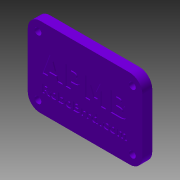
# Autodesk Inventor part: apmb_v1
Saved by Autodesk Inventor 2014 SP1 (Build 180222100, 222)
## iProperties
Created: 2014-02-28
Part Number: apmb_v1
Material: Generic
Document SubType Name: Modeling
Designer: Erin
Density: 1 g/cm^3
Appearance: Default
Author: Erin
Autodesk Inventor part; units mm, degrees
(part 1 of 13)
ref_plane "YZ Plane" through (0, 0, 0) normal (1, 0, 0) x (0, 1, 0)
ref_plane "XY Plane" through (0, 0, 0) normal (0, 0, 1) x (1, 0, 0)
sketch "Sketch1" plane through (0, 0, 0) normal (0, 1, 0) x (-1, 0, 0)
  line L0 (33.3312, 2.2987) -> (35.2468, 0.3832)
  line L1 (20.6882, 2.2987) -> (33.3312, 2.2987)
  line L2 (35.2468, 0.3832) -> (37.29, 0.3832)
  line L3 (22.987, 7.6623) -> (20.0497, 10.5996)
  line L4 (22.987, 2.2987) -> (22.987, 7.6623)
  line L5 (18.7727, 0.3832) -> (20.6882, 2.2987)
  line L6 (16.8571, 0.3832) -> (18.7727, 0.3832)
  line L7 (33.3312, 10.5996) -> (34.7358, 10.5996)
  line L8 (31.1601, 12.7705) -> (33.3312, 10.5996)
  spline S0 degree 3 poles (10.1653, 33.5866) (10.1653, 34.1226) (9.7308, 34.5571) (9.1948, 34.5571) knots 0 0 0 0 1 1 1 1
  line L9 (10.1653, 33.5866) -> (10.1653, 34.1226) construction
  line L10 (10.1653, 34.1226) -> (9.7308, 34.5571) construction
  line L11 (9.7308, 34.5571) -> (9.1948, 34.5571) construction
  spline S1 degree 3 poles (9.1948, 34.5571) (8.6588, 34.5571) (8.2242, 34.1226) (8.2242, 33.5866) knots 0 0 0 0 1 1 1 1
  line L12 (9.1948, 34.5571) -> (8.6588, 34.5571) construction
  line L13 (8.6588, 34.5571) -> (8.2242, 34.1226) construction
  line L14 (8.2242, 34.1226) -> (8.2242, 33.5866) construction
  spline S2 degree 3 poles (8.2242, 33.5866) (8.2242, 33.0506) (8.6588, 32.616) (9.1948, 32.616) knots 0 0 0 0 1 1 1 1
  line L15 (8.2242, 33.5866) -> (8.2242, 33.0506) construction
  line L16 (8.2242, 33.0506) -> (8.6588, 32.616) construction
  line L17 (8.6588, 32.616) -> (9.1948, 32.616) construction
  spline S3 degree 3 poles (9.1948, 32.616) (9.7308, 32.616) (10.1653, 33.0506) (10.1653, 33.5866) knots 0 0 0 0 1 1 1 1
  line L18 (9.1948, 32.616) -> (9.7308, 32.616) construction
  line L19 (9.7308, 32.616) -> (10.1653, 33.0506) construction
  line L20 (10.1653, 33.0506) -> (10.1653, 33.5866) construction
  spline S4 degree 3 poles (12.7194, 33.5866) (12.7194, 34.1226) (12.2849, 34.5571) (11.7489, 34.5571) knots 0 0 0 0 1 1 1 1
  line L21 (12.7194, 33.5866) -> (12.7194, 34.1226) construction
  line L22 (12.7194, 34.1226) -> (12.2849, 34.5571) construction
  line L23 (12.2849, 34.5571) -> (11.7489, 34.5571) construction
  spline S5 degree 3 poles (11.7489, 34.5571) (11.2129, 34.5571) (10.7783, 34.1226) (10.7783, 33.5866) knots 0 0 0 0 1 1 1 1
  line L24 (11.7489, 34.5571) -> (11.2129, 34.5571) construction
  line L25 (11.2129, 34.5571) -> (10.7783, 34.1226) construction
  line L26 (10.7783, 34.1226) -> (10.7783, 33.5866) construction
  spline S6 degree 3 poles (10.7783, 33.5866) (10.7783, 33.0506) (11.2129, 32.616) (11.7489, 32.616) knots 0 0 0 0 1 1 1 1
  line L27 (10.7783, 33.5866) -> (10.7783, 33.0506) construction
  line L28 (10.7783, 33.0506) -> (11.2129, 32.616) construction
  line L29 (11.2129, 32.616) -> (11.7489, 32.616) construction
  spline S7 degree 3 poles (11.7489, 32.616) (12.2849, 32.616) (12.7194, 33.0506) (12.7194, 33.5866) knots 0 0 0 0 1 1 1 1
  line L30 (11.7489, 32.616) -> (12.2849, 32.616) construction
  line L31 (12.2849, 32.616) -> (12.7194, 33.0506) construction
  line L32 (12.7194, 33.0506) -> (12.7194, 33.5866) construction
  spline S8 degree 3 poles (15.2735, 33.5866) (15.2735, 34.1226) (14.839, 34.5571) (14.303, 34.5571) knots 0 0 0 0 1 1 1 1
  line L33 (15.2735, 33.5866) -> (15.2735, 34.1226) construction
  line L34 (15.2735, 34.1226) -> (14.839, 34.5571) construction
  line L35 (14.839, 34.5571) -> (14.303, 34.5571) construction
  spline S9 degree 3 poles (14.303, 34.5571) (13.767, 34.5571) (13.3324, 34.1226) (13.3324, 33.5866) knots 0 0 0 0 1 1 1 1
  line L36 (14.303, 34.5571) -> (13.767, 34.5571) construction
  line L37 (13.767, 34.5571) -> (13.3324, 34.1226) construction
  line L38 (13.3324, 34.1226) -> (13.3324, 33.5866) construction
  spline S10 degree 3 poles (13.3324, 33.5866) (13.3324, 33.0506) (13.767, 32.616) (14.303, 32.616) knots 0 0 0 0 1 1 1 1
  line L39 (13.3324, 33.5866) -> (13.3324, 33.0506) construction
  line L40 (13.3324, 33.0506) -> (13.767, 32.616) construction
  line L41 (13.767, 32.616) -> (14.303, 32.616) construction
  spline S11 degree 3 poles (14.303, 32.616) (14.839, 32.616) (15.2735, 33.0506) (15.2735, 33.5866) knots 0 0 0 0 1 1 1 1
  line L42 (14.303, 32.616) -> (14.839, 32.616) construction
  line L43 (14.839, 32.616) -> (15.2735, 33.0506) construction
  line L44 (15.2735, 33.0506) -> (15.2735, 33.5866) construction
  spline S12 degree 3 poles (17.8276, 23.3701) (17.8276, 23.9061) (17.3931, 24.3407) (16.8571, 24.3407) knots 0 0 0 0 1 1 1 1
  line L45 (17.8276, 23.3701) -> (17.8276, 23.9061) construction
  line L46 (17.8276, 23.9061) -> (17.3931, 24.3407) construction
  line L47 (17.3931, 24.3407) -> (16.8571, 24.3407) construction
  spline S13 degree 3 poles (16.8571, 24.3407) (16.3211, 24.3407) (15.8866, 23.9061) (15.8866, 23.3701) knots 0 0 0 0 1 1 1 1
  line L48 (16.8571, 24.3407) -> (16.3211, 24.3407) construction
  line L49 (16.3211, 24.3407) -> (15.8866, 23.9061) construction
  line L50 (15.8866, 23.9061) -> (15.8866, 23.3701) construction
  spline S14 degree 3 poles (15.8866, 23.3701) (15.8866, 22.8341) (16.3211, 22.3996) (16.8571, 22.3996) knots 0 0 0 0 1 1 1 1
  line L51 (15.8866, 23.3701) -> (15.8866, 22.8341) construction
  line L52 (15.8866, 22.8341) -> (16.3211, 22.3996) construction
  line L53 (16.3211, 22.3996) -> (16.8571, 22.3996) construction
  spline S15 degree 3 poles (16.8571, 22.3996) (17.3931, 22.3996) (17.8276, 22.8341) (17.8276, 23.3701) knots 0 0 0 0 1 1 1 1
  line L54 (16.8571, 22.3996) -> (17.3931, 22.3996) construction
  line L55 (17.3931, 22.3996) -> (17.8276, 22.8341) construction
  line L56 (17.8276, 22.8341) -> (17.8276, 23.3701) construction
  spline S16 degree 3 poles (23.319, 22.2718) (23.319, 22.8078) (22.8844, 23.2424) (22.3485, 23.2424) knots 0 0 0 0 1 1 1 1
  line L57 (23.319, 22.2718) -> (23.319, 22.8078) construction
  line L58 (23.319, 22.8078) -> (22.8844, 23.2424) construction
  line L59 (22.8844, 23.2424) -> (22.3485, 23.2424) construction
  spline S17 degree 3 poles (22.3485, 23.2424) (21.8125, 23.2424) (21.3779, 22.8078) (21.3779, 22.2718) knots 0 0 0 0 1 1 1 1
  line L60 (22.3485, 23.2424) -> (21.8125, 23.2424) construction
  line L61 (21.8125, 23.2424) -> (21.3779, 22.8078) construction
  line L62 (21.3779, 22.8078) -> (21.3779, 22.2718) construction
  spline S18 degree 3 poles (21.3779, 22.2718) (21.3779, 21.7358) (21.8125, 21.3013) (22.3485, 21.3013) knots 0 0 0 0 1 1 1 1
  line L63 (21.3779, 22.2718) -> (21.3779, 21.7358) construction
  line L64 (21.3779, 21.7358) -> (21.8125, 21.3013) construction
  line L65 (21.8125, 21.3013) -> (22.3485, 21.3013) construction
  spline S19 degree 3 poles (22.3485, 21.3013) (22.8844, 21.3013) (23.319, 21.7358) (23.319, 22.2718) knots 0 0 0 0 1 1 1 1
  line L66 (22.3485, 21.3013) -> (22.8844, 21.3013) construction
  line L67 (22.8844, 21.3013) -> (23.319, 21.7358) construction
  line L68 (23.319, 21.7358) -> (23.319, 22.2718) construction
  spline S20 degree 3 poles (25.8731, 22.2718) (25.8731, 22.8078) (25.4385, 23.2424) (24.9026, 23.2424) knots 0 0 0 0 1 1 1 1
  line L69 (25.8731, 22.2718) -> (25.8731, 22.8078) construction
  line L70 (25.8731, 22.8078) -> (25.4385, 23.2424) construction
  line L71 (25.4385, 23.2424) -> (24.9026, 23.2424) construction
  spline S21 degree 3 poles (24.9026, 23.2424) (24.3666, 23.2424) (23.932, 22.8078) (23.932, 22.2718) knots 0 0 0 0 1 1 1 1
  line L72 (24.9026, 23.2424) -> (24.3666, 23.2424) construction
  line L73 (24.3666, 23.2424) -> (23.932, 22.8078) construction
  line L74 (23.932, 22.8078) -> (23.932, 22.2718) construction
  spline S22 degree 3 poles (23.932, 22.2718) (23.932, 21.7358) (24.3666, 21.3013) (24.9026, 21.3013) knots 0 0 0 0 1 1 1 1
  line L75 (23.932, 22.2718) -> (23.932, 21.7358) construction
  line L76 (23.932, 21.7358) -> (24.3666, 21.3013) construction
  line L77 (24.3666, 21.3013) -> (24.9026, 21.3013) construction
  spline S23 degree 3 poles (24.9026, 21.3013) (25.4385, 21.3013) (25.8731, 21.7358) (25.8731, 22.2718) knots 0 0 0 0 1 1 1 1
  line L78 (24.9026, 21.3013) -> (25.4385, 21.3013) construction
  line L79 (25.4385, 21.3013) -> (25.8731, 21.7358) construction
  line L80 (25.8731, 21.7358) -> (25.8731, 22.2718) construction
  spline S24 degree 3 poles (23.319, 24.8259) (23.319, 25.3619) (22.8844, 25.7965) (22.3485, 25.7965) knots 0 0 0 0 1 1 1 1
  line L81 (23.319, 24.8259) -> (23.319, 25.3619) construction
  line L82 (23.319, 25.3619) -> (22.8844, 25.7965) construction
  line L83 (22.8844, 25.7965) -> (22.3485, 25.7965) construction
  spline S25 degree 3 poles (22.3485, 25.7965) (21.8125, 25.7965) (21.3779, 25.3619) (21.3779, 24.8259) knots 0 0 0 0 1 1 1 1
  line L84 (22.3485, 25.7965) -> (21.8125, 25.7965) construction
  line L85 (21.8125, 25.7965) -> (21.3779, 25.3619) construction
  line L86 (21.3779, 25.3619) -> (21.3779, 24.8259) construction
  spline S26 degree 3 poles (21.3779, 24.8259) (21.3779, 24.2899) (21.8125, 23.8554) (22.3485, 23.8554) knots 0 0 0 0 1 1 1 1
  line L87 (21.3779, 24.8259) -> (21.3779, 24.2899) construction
  line L88 (21.3779, 24.2899) -> (21.8125, 23.8554) construction
  line L89 (21.8125, 23.8554) -> (22.3485, 23.8554) construction
  spline S27 degree 3 poles (22.3485, 23.8554) (22.8844, 23.8554) (23.319, 24.2899) (23.319, 24.8259) knots 0 0 0 0 1 1 1 1
  line L90 (22.3485, 23.8554) -> (22.8844, 23.8554) construction
  line L91 (22.8844, 23.8554) -> (23.319, 24.2899) construction
  line L92 (23.319, 24.2899) -> (23.319, 24.8259) construction
  spline S28 degree 3 poles (25.8731, 24.8259) (25.8731, 25.3619) (25.4385, 25.7965) (24.9026, 25.7965) knots 0 0 0 0 1 1 1 1
  line L93 (25.8731, 24.8259) -> (25.8731, 25.3619) construction
  line L94 (25.8731, 25.3619) -> (25.4385, 25.7965) construction
  line L95 (25.4385, 25.7965) -> (24.9026, 25.7965) construction
  spline S29 degree 3 poles (24.9026, 25.7965) (24.3666, 25.7965) (23.932, 25.3619) (23.932, 24.8259) knots 0 0 0 0 1 1 1 1
  line L96 (24.9026, 25.7965) -> (24.3666, 25.7965) construction
  line L97 (24.3666, 25.7965) -> (23.932, 25.3619) construction
  line L98 (23.932, 25.3619) -> (23.932, 24.8259) construction
  spline S30 degree 3 poles (23.932, 24.8259) (23.932, 24.2899) (24.3666, 23.8554) (24.9026, 23.8554) knots 0 0 0 0 1 1 1 1
  line L99 (23.932, 24.8259) -> (23.932, 24.2899) construction
  line L100 (23.932, 24.2899) -> (24.3666, 23.8554) construction
  line L101 (24.3666, 23.8554) -> (24.9026, 23.8554) construction
  spline S31 degree 3 poles (24.9026, 23.8554) (25.4385, 23.8554) (25.8731, 24.2899) (25.8731, 24.8259) knots 0 0 0 0 1 1 1 1
  line L102 (24.9026, 23.8554) -> (25.4385, 23.8554) construction
  line L103 (25.4385, 23.8554) -> (25.8731, 24.2899) construction
  line L104 (25.8731, 24.2899) -> (25.8731, 24.8259) construction
  spline S32 degree 3 poles (20.3818, 23.3701) (20.3818, 23.9061) (19.9472, 24.3407) (19.4112, 24.3407) knots 0 0 0 0 1 1 1 1
  line L105 (20.3818, 23.3701) -> (20.3818, 23.9061) construction
  line L106 (20.3818, 23.9061) -> (19.9472, 24.3407) construction
  line L107 (19.9472, 24.3407) -> (19.4112, 24.3407) construction
  spline S33 degree 3 poles (19.4112, 24.3407) (18.8752, 24.3407) (18.4407, 23.9061) (18.4407, 23.3701) knots 0 0 0 0 1 1 1 1
  line L108 (19.4112, 24.3407) -> (18.8752, 24.3407) construction
  line L109 (18.8752, 24.3407) -> (18.4407, 23.9061) construction
  line L110 (18.4407, 23.9061) -> (18.4407, 23.3701) construction
  spline S34 degree 3 poles (18.4407, 23.3701) (18.4407, 22.8341) (18.8752, 22.3996) (19.4112, 22.3996) knots 0 0 0 0 1 1 1 1
  line L111 (18.4407, 23.3701) -> (18.4407, 22.8341) construction
  line L112 (18.4407, 22.8341) -> (18.8752, 22.3996) construction
  line L113 (18.8752, 22.3996) -> (19.4112, 22.3996) construction
  spline S35 degree 3 poles (19.4112, 22.3996) (19.9472, 22.3996) (20.3818, 22.8341) (20.3818, 23.3701) knots 0 0 0 0 1 1 1 1
  line L114 (19.4112, 22.3996) -> (19.9472, 22.3996) construction
  line L115 (19.9472, 22.3996) -> (20.3818, 22.8341) construction
  line L116 (20.3818, 22.8341) -> (20.3818, 23.3701) construction
  spline S36 degree 3 poles (20.3818, 25.9242) (20.3818, 26.4602) (19.9472, 26.8948) (19.4112, 26.8948) knots 0 0 0 0 1 1 1 1
  line L117 (20.3818, 25.9242) -> (20.3818, 26.4602) construction
  line L118 (20.3818, 26.4602) -> (19.9472, 26.8948) construction
  line L119 (19.9472, 26.8948) -> (19.4112, 26.8948) construction
  spline S37 degree 3 poles (19.4112, 26.8948) (18.8752, 26.8948) (18.4407, 26.4602) (18.4407, 25.9242) knots 0 0 0 0 1 1 1 1
  line L120 (19.4112, 26.8948) -> (18.8752, 26.8948) construction
  line L121 (18.8752, 26.8948) -> (18.4407, 26.4602) construction
  line L122 (18.4407, 26.4602) -> (18.4407, 25.9242) construction
  spline S38 degree 3 poles (18.4407, 25.9242) (18.4407, 25.3882) (18.8752, 24.9537) (19.4112, 24.9537) knots 0 0 0 0 1 1 1 1
  line L123 (18.4407, 25.9242) -> (18.4407, 25.3882) construction
  line L124 (18.4407, 25.3882) -> (18.8752, 24.9537) construction
  line L125 (18.8752, 24.9537) -> (19.4112, 24.9537) construction
  spline S39 degree 3 poles (19.4112, 24.9537) (19.9472, 24.9537) (20.3818, 25.3882) (20.3818, 25.9242) knots 0 0 0 0 1 1 1 1
  line L126 (19.4112, 24.9537) -> (19.9472, 24.9537) construction
  line L127 (19.9472, 24.9537) -> (20.3818, 25.3882) construction
  line L128 (20.3818, 25.3882) -> (20.3818, 25.9242) construction
  spline S40 degree 3 poles (20.3818, 28.4784) (20.3818, 29.0143) (19.9472, 29.4489) (19.4112, 29.4489) knots 0 0 0 0 1 1 1 1
  line L129 (20.3818, 28.4784) -> (20.3818, 29.0143) construction
  line L130 (20.3818, 29.0143) -> (19.9472, 29.4489) construction
  line L131 (19.9472, 29.4489) -> (19.4112, 29.4489) construction
  spline S41 degree 3 poles (19.4112, 29.4489) (18.8752, 29.4489) (18.4407, 29.0143) (18.4407, 28.4784) knots 0 0 0 0 1 1 1 1
  line L132 (19.4112, 29.4489) -> (18.8752, 29.4489) construction
  line L133 (18.8752, 29.4489) -> (18.4407, 29.0143) construction
  line L134 (18.4407, 29.0143) -> (18.4407, 28.4784) construction
  spline S42 degree 3 poles (18.4407, 28.4784) (18.4407, 27.9423) (18.8752, 27.5078) (19.4112, 27.5078) knots 0 0 0 0 1 1 1 1
  line L135 (18.4407, 28.4784) -> (18.4407, 27.9423) construction
  line L136 (18.4407, 27.9423) -> (18.8752, 27.5078) construction
  line L137 (18.8752, 27.5078) -> (19.4112, 27.5078) construction
  spline S43 degree 3 poles (19.4112, 27.5078) (19.9472, 27.5078) (20.3818, 27.9423) (20.3818, 28.4784) knots 0 0 0 0 1 1 1 1
  line L138 (19.4112, 27.5078) -> (19.9472, 27.5078) construction
  line L139 (19.9472, 27.5078) -> (20.3818, 27.9423) construction
  line L140 (20.3818, 27.9423) -> (20.3818, 28.4784) construction
  spline S44 degree 3 poles (20.3818, 31.0325) (20.3818, 31.5684) (19.9472, 32.003) (19.4112, 32.003) knots 0 0 0 0 1 1 1 1
  line L141 (20.3818, 31.0325) -> (20.3818, 31.5684) construction
  line L142 (20.3818, 31.5684) -> (19.9472, 32.003) construction
  line L143 (19.9472, 32.003) -> (19.4112, 32.003) construction
  spline S45 degree 3 poles (19.4112, 32.003) (18.8752, 32.003) (18.4407, 31.5684) (18.4407, 31.0325) knots 0 0 0 0 1 1 1 1
  line L144 (19.4112, 32.003) -> (18.8752, 32.003) construction
  line L145 (18.8752, 32.003) -> (18.4407, 31.5684) construction
  line L146 (18.4407, 31.5684) -> (18.4407, 31.0325) construction
  spline S46 degree 3 poles (18.4407, 31.0325) (18.4407, 30.4965) (18.8752, 30.0619) (19.4112, 30.0619) knots 0 0 0 0 1 1 1 1
  line L147 (18.4407, 31.0325) -> (18.4407, 30.4965) construction
  line L148 (18.4407, 30.4965) -> (18.8752, 30.0619) construction
  line L149 (18.8752, 30.0619) -> (19.4112, 30.0619) construction
  spline S47 degree 3 poles (19.4112, 30.0619) (19.9472, 30.0619) (20.3818, 30.4965) (20.3818, 31.0325) knots 0 0 0 0 1 1 1 1
  line L150 (19.4112, 30.0619) -> (19.9472, 30.0619) construction
  line L151 (19.9472, 30.0619) -> (20.3818, 30.4965) construction
  line L152 (20.3818, 30.4965) -> (20.3818, 31.0325) construction
  spline S48 degree 3 poles (17.8276, 25.9242) (17.8276, 26.4602) (17.3931, 26.8948) (16.8571, 26.8948) knots 0 0 0 0 1 1 1 1
  line L153 (17.8276, 25.9242) -> (17.8276, 26.4602) construction
  line L154 (17.8276, 26.4602) -> (17.3931, 26.8948) construction
  line L155 (17.3931, 26.8948) -> (16.8571, 26.8948) construction
  spline S49 degree 3 poles (16.8571, 26.8948) (16.3211, 26.8948) (15.8866, 26.4602) (15.8866, 25.9242) knots 0 0 0 0 1 1 1 1
  line L156 (16.8571, 26.8948) -> (16.3211, 26.8948) construction
  line L157 (16.3211, 26.8948) -> (15.8866, 26.4602) construction
  line L158 (15.8866, 26.4602) -> (15.8866, 25.9242) construction
  spline S50 degree 3 poles (15.8866, 25.9242) (15.8866, 25.3882) (16.3211, 24.9537) (16.8571, 24.9537) knots 0 0 0 0 1 1 1 1
  line L159 (15.8866, 25.9242) -> (15.8866, 25.3882) construction
  line L160 (15.8866, 25.3882) -> (16.3211, 24.9537) construction
  line L161 (16.3211, 24.9537) -> (16.8571, 24.9537) construction
  spline S51 degree 3 poles (16.8571, 24.9537) (17.3931, 24.9537) (17.8276, 25.3882) (17.8276, 25.9242) knots 0 0 0 0 1 1 1 1
  line L162 (16.8571, 24.9537) -> (17.3931, 24.9537) construction
  line L163 (17.3931, 24.9537) -> (17.8276, 25.3882) construction
  line L164 (17.8276, 25.3882) -> (17.8276, 25.9242) construction
  spline S52 degree 3 poles (17.8276, 28.4784) (17.8276, 29.0143) (17.3931, 29.4489) (16.8571, 29.4489) knots 0 0 0 0 1 1 1 1
  line L165 (17.8276, 28.4784) -> (17.8276, 29.0143) construction
  line L166 (17.8276, 29.0143) -> (17.3931, 29.4489) construction
  line L167 (17.3931, 29.4489) -> (16.8571, 29.4489) construction
  spline S53 degree 3 poles (16.8571, 29.4489) (16.3211, 29.4489) (15.8866, 29.0143) (15.8866, 28.4784) knots 0 0 0 0 1 1 1 1
  line L168 (16.8571, 29.4489) -> (16.3211, 29.4489) construction
  line L169 (16.3211, 29.4489) -> (15.8866, 29.0143) construction
  line L170 (15.8866, 29.0143) -> (15.8866, 28.4784) construction
  spline S54 degree 3 poles (15.8866, 28.4784) (15.8866, 27.9423) (16.3211, 27.5078) (16.8571, 27.5078) knots 0 0 0 0 1 1 1 1
  line L171 (15.8866, 28.4784) -> (15.8866, 27.9423) construction
  line L172 (15.8866, 27.9423) -> (16.3211, 27.5078) construction
  line L173 (16.3211, 27.5078) -> (16.8571, 27.5078) construction
  spline S55 degree 3 poles (16.8571, 27.5078) (17.3931, 27.5078) (17.8276, 27.9423) (17.8276, 28.4784) knots 0 0 0 0 1 1 1 1
  line L174 (16.8571, 27.5078) -> (17.3931, 27.5078) construction
  line L175 (17.3931, 27.5078) -> (17.8276, 27.9423) construction
  line L176 (17.8276, 27.9423) -> (17.8276, 28.4784) construction
  spline S56 degree 3 poles (17.8276, 31.0325) (17.8276, 31.5684) (17.3931, 32.003) (16.8571, 32.003) knots 0 0 0 0 1 1 1 1
  line L177 (17.8276, 31.0325) -> (17.8276, 31.5684) construction
  line L178 (17.8276, 31.5684) -> (17.3931, 32.003) construction
  line L179 (17.3931, 32.003) -> (16.8571, 32.003) construction
  spline S57 degree 3 poles (16.8571, 32.003) (16.3211, 32.003) (15.8866, 31.5684) (15.8866, 31.0325) knots 0 0 0 0 1 1 1 1
  line L180 (16.8571, 32.003) -> (16.3211, 32.003) construction
  line L181 (16.3211, 32.003) -> (15.8866, 31.5684) construction
  line L182 (15.8866, 31.5684) -> (15.8866, 31.0325) construction
  spline S58 degree 3 poles (15.8866, 31.0325) (15.8866, 30.4965) (16.3211, 30.0619) (16.8571, 30.0619) knots 0 0 0 0 1 1 1 1
  line L183 (15.8866, 31.0325) -> (15.8866, 30.4965) construction
  line L184 (15.8866, 30.4965) -> (16.3211, 30.0619) construction
  line L185 (16.3211, 30.0619) -> (16.8571, 30.0619) construction
  spline S59 degree 3 poles (16.8571, 30.0619) (17.3931, 30.0619) (17.8276, 30.4965) (17.8276, 31.0325) knots 0 0 0 0 1 1 1 1
  line L186 (16.8571, 30.0619) -> (17.3931, 30.0619) construction
  line L187 (17.3931, 30.0619) -> (17.8276, 30.4965) construction
  line L188 (17.8276, 30.4965) -> (17.8276, 31.0325) construction
  spline S60 degree 3 poles (38.2606, 33.5866) (38.2606, 34.1226) (37.826, 34.5571) (37.29, 34.5571) knots 0 0 0 0 1 1 1 1
  line L189 (38.2606, 33.5866) -> (38.2606, 34.1226) construction
  line L190 (38.2606, 34.1226) -> (37.826, 34.5571) construction
  line L191 (37.826, 34.5571) -> (37.29, 34.5571) construction
  spline S61 degree 3 poles (37.29, 34.5571) (36.754, 34.5571) (36.3194, 34.1226) (36.3194, 33.5866) knots 0 0 0 0 1 1 1 1
  line L192 (37.29, 34.5571) -> (36.754, 34.5571) construction
  line L193 (36.754, 34.5571) -> (36.3194, 34.1226) construction
  line L194 (36.3194, 34.1226) -> (36.3194, 33.5866) construction
  spline S62 degree 3 poles (36.3194, 33.5866) (36.3194, 33.0506) (36.754, 32.616) (37.29, 32.616) knots 0 0 0 0 1 1 1 1
  line L195 (36.3194, 33.5866) -> (36.3194, 33.0506) construction
  line L196 (36.3194, 33.0506) -> (36.754, 32.616) construction
  line L197 (36.754, 32.616) -> (37.29, 32.616) construction
  spline S63 degree 3 poles (37.29, 32.616) (37.826, 32.616) (38.2606, 33.0506) (38.2606, 33.5866) knots 0 0 0 0 1 1 1 1
  line L198 (37.29, 32.616) -> (37.826, 32.616) construction
  line L199 (37.826, 32.616) -> (38.2606, 33.0506) construction
  line L200 (38.2606, 33.0506) -> (38.2606, 33.5866) construction
  spline S64 degree 3 poles (40.8147, 33.5866) (40.8147, 34.1226) (40.3801, 34.5571) (39.8441, 34.5571) knots 0 0 0 0 1 1 1 1
  line L201 (40.8147, 33.5866) -> (40.8147, 34.1226) construction
  line L202 (40.8147, 34.1226) -> (40.3801, 34.5571) construction
  line L203 (40.3801, 34.5571) -> (39.8441, 34.5571) construction
  spline S65 degree 3 poles (39.8441, 34.5571) (39.3081, 34.5571) (38.8735, 34.1226) (38.8735, 33.5866) knots 0 0 0 0 1 1 1 1
  line L204 (39.8441, 34.5571) -> (39.3081, 34.5571) construction
  line L205 (39.3081, 34.5571) -> (38.8735, 34.1226) construction
  line L206 (38.8735, 34.1226) -> (38.8735, 33.5866) construction
  spline S66 degree 3 poles (38.8735, 33.5866) (38.8735, 33.0506) (39.3081, 32.616) (39.8441, 32.616) knots 0 0 0 0 1 1 1 1
  line L207 (38.8735, 33.5866) -> (38.8735, 33.0506) construction
  line L208 (38.8735, 33.0506) -> (39.3081, 32.616) construction
  line L209 (39.3081, 32.616) -> (39.8441, 32.616) construction
  spline S67 degree 3 poles (39.8441, 32.616) (40.3801, 32.616) (40.8147, 33.0506) (40.8147, 33.5866) knots 0 0 0 0 1 1 1 1
  line L210 (39.8441, 32.616) -> (40.3801, 32.616) construction
  line L211 (40.3801, 32.616) -> (40.8147, 33.0506) construction
  line L212 (40.8147, 33.0506) -> (40.8147, 33.5866) construction
  spline S68 degree 3 poles (43.3688, 33.5866) (43.3688, 34.1226) (42.9342, 34.5571) (42.3982, 34.5571) knots 0 0 0 0 1 1 1 1
  line L213 (43.3688, 33.5866) -> (43.3688, 34.1226) construction
  line L214 (43.3688, 34.1226) -> (42.9342, 34.5571) construction
  line L215 (42.9342, 34.5571) -> (42.3982, 34.5571) construction
  spline S69 degree 3 poles (42.3982, 34.5571) (41.8622, 34.5571) (41.4277, 34.1226) (41.4277, 33.5866) knots 0 0 0 0 1 1 1 1
  line L216 (42.3982, 34.5571) -> (41.8622, 34.5571) construction
  line L217 (41.8622, 34.5571) -> (41.4277, 34.1226) construction
  line L218 (41.4277, 34.1226) -> (41.4277, 33.5866) construction
  spline S70 degree 3 poles (41.4277, 33.5866) (41.4277, 33.0506) (41.8622, 32.616) (42.3982, 32.616) knots 0 0 0 0 1 1 1 1
  line L219 (41.4277, 33.5866) -> (41.4277, 33.0506) construction
  line L220 (41.4277, 33.0506) -> (41.8622, 32.616) construction
  line L221 (41.8622, 32.616) -> (42.3982, 32.616) construction
  spline S71 degree 3 poles (42.3982, 32.616) (42.9342, 32.616) (43.3688, 33.0506) (43.3688, 33.5866) knots 0 0 0 0 1 1 1 1
  line L222 (42.3982, 32.616) -> (42.9342, 32.616) construction
  line L223 (42.9342, 32.616) -> (43.3688, 33.0506) construction
  line L224 (43.3688, 33.0506) -> (43.3688, 33.5866) construction
  spline S72 degree 3 poles (45.9229, 33.5866) (45.9229, 34.1226) (45.4883, 34.5571) (44.9523, 34.5571) knots 0 0 0 0 1 1 1 1
  line L225 (45.9229, 33.5866) -> (45.9229, 34.1226) construction
  line L226 (45.9229, 34.1226) -> (45.4883, 34.5571) construction
  line L227 (45.4883, 34.5571) -> (44.9523, 34.5571) construction
  spline S73 degree 3 poles (44.9523, 34.5571) (44.4163, 34.5571) (43.9818, 34.1226) (43.9818, 33.5866) knots 0 0 0 0 1 1 1 1
  line L228 (44.9523, 34.5571) -> (44.4163, 34.5571) construction
  line L229 (44.4163, 34.5571) -> (43.9818, 34.1226) construction
  line L230 (43.9818, 34.1226) -> (43.9818, 33.5866) construction
  spline S74 degree 3 poles (43.9818, 33.5866) (43.9818, 33.0506) (44.4163, 32.616) (44.9523, 32.616) knots 0 0 0 0 1 1 1 1
  line L231 (43.9818, 33.5866) -> (43.9818, 33.0506) construction
  line L232 (43.9818, 33.0506) -> (44.4163, 32.616) construction
  line L233 (44.4163, 32.616) -> (44.9523, 32.616) construction
  spline S75 degree 3 poles (44.9523, 32.616) (45.4883, 32.616) (45.9229, 33.0506) (45.9229, 33.5866) knots 0 0 0 0 1 1 1 1
  line L234 (44.9523, 32.616) -> (45.4883, 32.616) construction
  line L235 (45.4883, 32.616) -> (45.9229, 33.0506) construction
  line L236 (45.9229, 33.0506) -> (45.9229, 33.5866) construction
  spline S76 degree 3 poles (34.4294, 0.3832) (34.4294, 0.9191) (33.9948, 1.3537) (33.4588, 1.3537) knots 0 0 0 0 1 1 1 1
  line L237 (34.4294, 0.3832) -> (34.4294, 0.9191) construction
  line L238 (34.4294, 0.9191) -> (33.9948, 1.3537) construction
  line L239 (33.9948, 1.3537) -> (33.4588, 1.3537) construction
  spline S77 degree 3 poles (33.4588, 1.3537) (32.9228, 1.3537) (32.4883, 0.9191) (32.4883, 0.3832) knots 0 0 0 0 1 1 1 1
  line L240 (33.4588, 1.3537) -> (32.9228, 1.3537) construction
  line L241 (32.9228, 1.3537) -> (32.4883, 0.9191) construction
  line L242 (32.4883, 0.9191) -> (32.4883, 0.3832) construction
  spline S78 degree 3 poles (32.4883, 0.3832) (32.4883, -0.1529) (32.9228, -0.5874) (33.4588, -0.5874) knots 0 0 0 0 1 1 1 1
  line L243 (32.4883, 0.3832) -> (32.4883, -0.1529) construction
  line L244 (32.4883, -0.1529) -> (32.9228, -0.5874) construction
  line L245 (32.9228, -0.5874) -> (33.4588, -0.5874) construction
  spline S79 degree 3 poles (33.4588, -0.5874) (33.9948, -0.5874) (34.4294, -0.1529) (34.4294, 0.3832) knots 0 0 0 0 1 1 1 1
  line L246 (33.4588, -0.5874) -> (33.9948, -0.5874) construction
  line L247 (33.9948, -0.5874) -> (34.4294, -0.1529) construction
  line L248 (34.4294, -0.1529) -> (34.4294, 0.3832) construction
  spline S80 degree 3 poles (31.8752, 0.3832) (31.8752, 0.9191) (31.4407, 1.3537) (30.9047, 1.3537) knots 0 0 0 0 1 1 1 1
  line L249 (31.8752, 0.3832) -> (31.8752, 0.9191) construction
  line L250 (31.8752, 0.9191) -> (31.4407, 1.3537) construction
  line L251 (31.4407, 1.3537) -> (30.9047, 1.3537) construction
  spline S81 degree 3 poles (30.9047, 1.3537) (30.3687, 1.3537) (29.9342, 0.9191) (29.9342, 0.3832) knots 0 0 0 0 1 1 1 1
  line L252 (30.9047, 1.3537) -> (30.3687, 1.3537) construction
  line L253 (30.3687, 1.3537) -> (29.9342, 0.9191) construction
  line L254 (29.9342, 0.9191) -> (29.9342, 0.3832) construction
  spline S82 degree 3 poles (29.9342, 0.3832) (29.9342, -0.1529) (30.3687, -0.5874) (30.9047, -0.5874) knots 0 0 0 0 1 1 1 1
  line L255 (29.9342, 0.3832) -> (29.9342, -0.1529) construction
  line L256 (29.9342, -0.1529) -> (30.3687, -0.5874) construction
  line L257 (30.3687, -0.5874) -> (30.9047, -0.5874) construction
  spline S83 degree 3 poles (30.9047, -0.5874) (31.4407, -0.5874) (31.8752, -0.1529) (31.8752, 0.3832) knots 0 0 0 0 1 1 1 1
  line L258 (30.9047, -0.5874) -> (31.4407, -0.5874) construction
  line L259 (31.4407, -0.5874) -> (31.8752, -0.1529) construction
  line L260 (31.8752, -0.1529) -> (31.8752, 0.3832) construction
  spline S84 degree 3 poles (29.3211, 0.3832) (29.3211, 0.9191) (28.8866, 1.3537) (28.3506, 1.3537) knots 0 0 0 0 1 1 1 1
  line L261 (29.3211, 0.3832) -> (29.3211, 0.9191) construction
  line L262 (29.3211, 0.9191) -> (28.8866, 1.3537) construction
  line L263 (28.8866, 1.3537) -> (28.3506, 1.3537) construction
  spline S85 degree 3 poles (28.3506, 1.3537) (27.8146, 1.3537) (27.3801, 0.9191) (27.3801, 0.3832) knots 0 0 0 0 1 1 1 1
  line L264 (28.3506, 1.3537) -> (27.8146, 1.3537) construction
  line L265 (27.8146, 1.3537) -> (27.3801, 0.9191) construction
  line L266 (27.3801, 0.9191) -> (27.3801, 0.3832) construction
  spline S86 degree 3 poles (27.3801, 0.3832) (27.3801, -0.1529) (27.8146, -0.5874) (28.3506, -0.5874) knots 0 0 0 0 1 1 1 1
  line L267 (27.3801, 0.3832) -> (27.3801, -0.1529) construction
  line L268 (27.3801, -0.1529) -> (27.8146, -0.5874) construction
  line L269 (27.8146, -0.5874) -> (28.3506, -0.5874) construction
  spline S87 degree 3 poles (28.3506, -0.5874) (28.8866, -0.5874) (29.3211, -0.1529) (29.3211, 0.3832) knots 0 0 0 0 1 1 1 1
  line L270 (28.3506, -0.5874) -> (28.8866, -0.5874) construction
  line L271 (28.8866, -0.5874) -> (29.3211, -0.1529) construction
  line L272 (29.3211, -0.1529) -> (29.3211, 0.3832) construction
  spline S88 degree 3 poles (43.3688, 0.3832) (43.3688, 0.9191) (42.9342, 1.3537) (42.3982, 1.3537) knots 0 0 0 0 1 1 1 1
  line L273 (43.3688, 0.3832) -> (43.3688, 0.9191) construction
  line L274 (43.3688, 0.9191) -> (42.9342, 1.3537) construction
  line L275 (42.9342, 1.3537) -> (42.3982, 1.3537) construction
  spline S89 degree 3 poles (42.3982, 1.3537) (41.8622, 1.3537) (41.4277, 0.9191) (41.4277, 0.3832) knots 0 0 0 0 1 1 1 1
  line L276 (42.3982, 1.3537) -> (41.8622, 1.3537) construction
  line L277 (41.8622, 1.3537) -> (41.4277, 0.9191) construction
  line L278 (41.4277, 0.9191) -> (41.4277, 0.3832) construction
  spline S90 degree 3 poles (41.4277, 0.3832) (41.4277, -0.1529) (41.8622, -0.5874) (42.3982, -0.5874) knots 0 0 0 0 1 1 1 1
  line L279 (41.4277, 0.3832) -> (41.4277, -0.1529) construction
  line L280 (41.4277, -0.1529) -> (41.8622, -0.5874) construction
  line L281 (41.8622, -0.5874) -> (42.3982, -0.5874) construction
  spline S91 degree 3 poles (42.3982, -0.5874) (42.9342, -0.5874) (43.3688, -0.1529) (43.3688, 0.3832) knots 0 0 0 0 1 1 1 1
  line L282 (42.3982, -0.5874) -> (42.9342, -0.5874) construction
  line L283 (42.9342, -0.5874) -> (43.3688, -0.1529) construction
  line L284 (43.3688, -0.1529) -> (43.3688, 0.3832) construction
  spline S92 degree 3 poles (35.7064, 2.9373) (35.7064, 3.4732) (35.2719, 3.9078) (34.7358, 3.9078) knots 0 0 0 0 1 1 1 1
  line L285 (35.7064, 2.9373) -> (35.7064, 3.4732) construction
  line L286 (35.7064, 3.4732) -> (35.2719, 3.9078) construction
  line L287 (35.2719, 3.9078) -> (34.7358, 3.9078) construction
  spline S93 degree 3 poles (34.7358, 3.9078) (34.1999, 3.9078) (33.7653, 3.4732) (33.7653, 2.9373) knots 0 0 0 0 1 1 1 1
  line L288 (34.7358, 3.9078) -> (34.1999, 3.9078) construction
  line L289 (34.1999, 3.9078) -> (33.7653, 3.4732) construction
  line L290 (33.7653, 3.4732) -> (33.7653, 2.9373) construction
  spline S94 degree 3 poles (33.7653, 2.9373) (33.7653, 2.4013) (34.1999, 1.9667) (34.7358, 1.9667) knots 0 0 0 0 1 1 1 1
  line L291 (33.7653, 2.9373) -> (33.7653, 2.4013) construction
  line L292 (33.7653, 2.4013) -> (34.1999, 1.9667) construction
  line L293 (34.1999, 1.9667) -> (34.7358, 1.9667) construction
  spline S95 degree 3 poles (34.7358, 1.9667) (35.2719, 1.9667) (35.7064, 2.4013) (35.7064, 2.9373) knots 0 0 0 0 1 1 1 1
  line L294 (34.7358, 1.9667) -> (35.2719, 1.9667) construction
  line L295 (35.2719, 1.9667) -> (35.7064, 2.4013) construction
  line L296 (35.7064, 2.4013) -> (35.7064, 2.9373) construction
  spline S96 degree 3 poles (35.7064, 5.4914) (35.7064, 6.0273) (35.2719, 6.4619) (34.7358, 6.4619) knots 0 0 0 0 1 1 1 1
  line L297 (35.7064, 5.4914) -> (35.7064, 6.0273) construction
  line L298 (35.7064, 6.0273) -> (35.2719, 6.4619) construction
  line L299 (35.2719, 6.4619) -> (34.7358, 6.4619) construction
  spline S97 degree 3 poles (34.7358, 6.4619) (34.1999, 6.4619) (33.7653, 6.0273) (33.7653, 5.4914) knots 0 0 0 0 1 1 1 1
  line L300 (34.7358, 6.4619) -> (34.1999, 6.4619) construction
  line L301 (34.1999, 6.4619) -> (33.7653, 6.0273) construction
  line L302 (33.7653, 6.0273) -> (33.7653, 5.4914) construction
  spline S98 degree 3 poles (33.7653, 5.4914) (33.7653, 4.9554) (34.1999, 4.5208) (34.7358, 4.5208) knots 0 0 0 0 1 1 1 1
  line L303 (33.7653, 5.4914) -> (33.7653, 4.9554) construction
  line L304 (33.7653, 4.9554) -> (34.1999, 4.5208) construction
  line L305 (34.1999, 4.5208) -> (34.7358, 4.5208) construction
  spline S99 degree 3 poles (34.7358, 4.5208) (35.2719, 4.5208) (35.7064, 4.9554) (35.7064, 5.4914) knots 0 0 0 0 1 1 1 1
  line L306 (34.7358, 4.5208) -> (35.2719, 4.5208) construction
  line L307 (35.2719, 4.5208) -> (35.7064, 4.9554) construction
  line L308 (35.7064, 4.9554) -> (35.7064, 5.4914) construction
  spline S100 degree 3 poles (38.2606, 5.4914) (38.2606, 6.0273) (37.826, 6.4619) (37.29, 6.4619) knots 0 0 0 0 1 1 1 1
  line L309 (38.2606, 5.4914) -> (38.2606, 6.0273) construction
  line L310 (38.2606, 6.0273) -> (37.826, 6.4619) construction
  line L311 (37.826, 6.4619) -> (37.29, 6.4619) construction
  spline S101 degree 3 poles (37.29, 6.4619) (36.754, 6.4619) (36.3194, 6.0273) (36.3194, 5.4914) knots 0 0 0 0 1 1 1 1
  line L312 (37.29, 6.4619) -> (36.754, 6.4619) construction
  line L313 (36.754, 6.4619) -> (36.3194, 6.0273) construction
  line L314 (36.3194, 6.0273) -> (36.3194, 5.4914) construction
  spline S102 degree 3 poles (36.3194, 5.4914) (36.3194, 4.9554) (36.754, 4.5208) (37.29, 4.5208) knots 0 0 0 0 1 1 1 1
  line L315 (36.3194, 5.4914) -> (36.3194, 4.9554) construction
  line L316 (36.3194, 4.9554) -> (36.754, 4.5208) construction
  line L317 (36.754, 4.5208) -> (37.29, 4.5208) construction
  spline S103 degree 3 poles (37.29, 4.5208) (37.826, 4.5208) (38.2606, 4.9554) (38.2606, 5.4914) knots 0 0 0 0 1 1 1 1
  line L318 (37.29, 4.5208) -> (37.826, 4.5208) construction
  line L319 (37.826, 4.5208) -> (38.2606, 4.9554) construction
  line L320 (38.2606, 4.9554) -> (38.2606, 5.4914) construction
  spline S104 degree 3 poles (38.2606, 0.3832) (38.2606, 0.9191) (37.826, 1.3537) (37.29, 1.3537) knots 0 0 0 0 1 1 1 1
  line L321 (38.2606, 0.3832) -> (38.2606, 0.9191) construction
  line L322 (38.2606, 0.9191) -> (37.826, 1.3537) construction
  line L323 (37.826, 1.3537) -> (37.29, 1.3537) construction
  spline S105 degree 3 poles (37.29, 1.3537) (36.754, 1.3537) (36.3194, 0.9191) (36.3194, 0.3832) knots 0 0 0 0 1 1 1 1
  line L324 (37.29, 1.3537) -> (36.754, 1.3537) construction
  line L325 (36.754, 1.3537) -> (36.3194, 0.9191) construction
  line L326 (36.3194, 0.9191) -> (36.3194, 0.3832) construction
  spline S106 degree 3 poles (36.3194, 0.3832) (36.3194, -0.1529) (36.754, -0.5874) (37.29, -0.5874) knots 0 0 0 0 1 1 1 1
  line L327 (36.3194, 0.3832) -> (36.3194, -0.1529) construction
  line L328 (36.3194, -0.1529) -> (36.754, -0.5874) construction
  line L329 (36.754, -0.5874) -> (37.29, -0.5874) construction
  spline S107 degree 3 poles (37.29, -0.5874) (37.826, -0.5874) (38.2606, -0.1529) (38.2606, 0.3832) knots 0 0 0 0 1 1 1 1
  line L330 (37.29, -0.5874) -> (37.826, -0.5874) construction
  line L331 (37.826, -0.5874) -> (38.2606, -0.1529) construction
  line L332 (38.2606, -0.1529) -> (38.2606, 0.3832) construction
  spline S108 degree 3 poles (40.8147, 0.3832) (40.8147, 0.9191) (40.3801, 1.3537) (39.8441, 1.3537) knots 0 0 0 0 1 1 1 1
  line L333 (40.8147, 0.3832) -> (40.8147, 0.9191) construction
  line L334 (40.8147, 0.9191) -> (40.3801, 1.3537) construction
  line L335 (40.3801, 1.3537) -> (39.8441, 1.3537) construction
  spline S109 degree 3 poles (39.8441, 1.3537) (39.3081, 1.3537) (38.8735, 0.9191) (38.8735, 0.3832) knots 0 0 0 0 1 1 1 1
  line L336 (39.8441, 1.3537) -> (39.3081, 1.3537) construction
  line L337 (39.3081, 1.3537) -> (38.8735, 0.9191) construction
  line L338 (38.8735, 0.9191) -> (38.8735, 0.3832) construction
  spline S110 degree 3 poles (38.8735, 0.3832) (38.8735, -0.1529) (39.3081, -0.5874) (39.8441, -0.5874) knots 0 0 0 0 1 1 1 1
  line L339 (38.8735, 0.3832) -> (38.8735, -0.1529) construction
  line L340 (38.8735, -0.1529) -> (39.3081, -0.5874) construction
  line L341 (39.3081, -0.5874) -> (39.8441, -0.5874) construction
  spline S111 degree 3 poles (39.8441, -0.5874) (40.3801, -0.5874) (40.8147, -0.1529) (40.8147, 0.3832) knots 0 0 0 0 1 1 1 1
  line L342 (39.8441, -0.5874) -> (40.3801, -0.5874) construction
  line L343 (40.3801, -0.5874) -> (40.8147, -0.1529) construction
  line L344 (40.8147, -0.1529) -> (40.8147, 0.3832) construction
  spline S112 degree 3 poles (38.2606, 2.9373) (38.2606, 3.4732) (37.826, 3.9078) (37.29, 3.9078) knots 0 0 0 0 1 1 1 1
  line L345 (38.2606, 2.9373) -> (38.2606, 3.4732) construction
  line L346 (38.2606, 3.4732) -> (37.826, 3.9078) construction
  line L347 (37.826, 3.9078) -> (37.29, 3.9078) construction
  spline S113 degree 3 poles (37.29, 3.9078) (36.754, 3.9078) (36.3194, 3.4732) (36.3194, 2.9373) knots 0 0 0 0 1 1 1 1
  line L348 (37.29, 3.9078) -> (36.754, 3.9078) construction
  line L349 (36.754, 3.9078) -> (36.3194, 3.4732) construction
  line L350 (36.3194, 3.4732) -> (36.3194, 2.9373) construction
  spline S114 degree 3 poles (36.3194, 2.9373) (36.3194, 2.4013) (36.754, 1.9667) (37.29, 1.9667) knots 0 0 0 0 1 1 1 1
  line L351 (36.3194, 2.9373) -> (36.3194, 2.4013) construction
  line L352 (36.3194, 2.4013) -> (36.754, 1.9667) construction
  line L353 (36.754, 1.9667) -> (37.29, 1.9667) construction
  spline S115 degree 3 poles (37.29, 1.9667) (37.826, 1.9667) (38.2606, 2.4013) (38.2606, 2.9373) knots 0 0 0 0 1 1 1 1
  line L354 (37.29, 1.9667) -> (37.826, 1.9667) construction
  line L355 (37.826, 1.9667) -> (38.2606, 2.4013) construction
  line L356 (38.2606, 2.4013) -> (38.2606, 2.9373) construction
  spline S116 degree 3 poles (35.7064, 8.0455) (35.7064, 8.5815) (35.2719, 9.016) (34.7358, 9.016) knots 0 0 0 0 1 1 1 1
  line L357 (35.7064, 8.0455) -> (35.7064, 8.5815) construction
  line L358 (35.7064, 8.5815) -> (35.2719, 9.016) construction
  line L359 (35.2719, 9.016) -> (34.7358, 9.016) construction
  spline S117 degree 3 poles (34.7358, 9.016) (34.1999, 9.016) (33.7653, 8.5815) (33.7653, 8.0455) knots 0 0 0 0 1 1 1 1
  line L360 (34.7358, 9.016) -> (34.1999, 9.016) construction
  line L361 (34.1999, 9.016) -> (33.7653, 8.5815) construction
  line L362 (33.7653, 8.5815) -> (33.7653, 8.0455) construction
  spline S118 degree 3 poles (33.7653, 8.0455) (33.7653, 7.5095) (34.1999, 7.0749) (34.7358, 7.0749) knots 0 0 0 0 1 1 1 1
  line L363 (33.7653, 8.0455) -> (33.7653, 7.5095) construction
  line L364 (33.7653, 7.5095) -> (34.1999, 7.0749) construction
  line L365 (34.1999, 7.0749) -> (34.7358, 7.0749) construction
  spline S119 degree 3 poles (34.7358, 7.0749) (35.2719, 7.0749) (35.7064, 7.5095) (35.7064, 8.0455) knots 0 0 0 0 1 1 1 1
  line L366 (34.7358, 7.0749) -> (35.2719, 7.0749) construction
  line L367 (35.2719, 7.0749) -> (35.7064, 7.5095) construction
  line L368 (35.7064, 7.5095) -> (35.7064, 8.0455) construction
  spline S120 degree 3 poles (38.2606, 8.0455) (38.2606, 8.5815) (37.826, 9.016) (37.29, 9.016) knots 0 0 0 0 1 1 1 1
  line L369 (38.2606, 8.0455) -> (38.2606, 8.5815) construction
  line L370 (38.2606, 8.5815) -> (37.826, 9.016) construction
  line L371 (37.826, 9.016) -> (37.29, 9.016) construction
  spline S121 degree 3 poles (37.29, 9.016) (36.754, 9.016) (36.3194, 8.5815) (36.3194, 8.0455) knots 0 0 0 0 1 1 1 1
  line L372 (37.29, 9.016) -> (36.754, 9.016) construction
  line L373 (36.754, 9.016) -> (36.3194, 8.5815) construction
  line L374 (36.3194, 8.5815) -> (36.3194, 8.0455) construction
  spline S122 degree 3 poles (36.3194, 8.0455) (36.3194, 7.5095) (36.754, 7.0749) (37.29, 7.0749) knots 0 0 0 0 1 1 1 1
  line L375 (36.3194, 8.0455) -> (36.3194, 7.5095) construction
  line L376 (36.3194, 7.5095) -> (36.754, 7.0749) construction
  line L377 (36.754, 7.0749) -> (37.29, 7.0749) construction
  spline S123 degree 3 poles (37.29, 7.0749) (37.826, 7.0749) (38.2606, 7.5095) (38.2606, 8.0455) knots 0 0 0 0 1 1 1 1
  line L378 (37.29, 7.0749) -> (37.826, 7.0749) construction
  line L379 (37.826, 7.0749) -> (38.2606, 7.5095) construction
  line L380 (38.2606, 7.5095) -> (38.2606, 8.0455) construction
  spline S124 degree 3 poles (35.7064, 10.5996) (35.7064, 11.1356) (35.2719, 11.5701) (34.7358, 11.5701) knots 0 0 0 0 1 1 1 1
  line L381 (35.7064, 10.5996) -> (35.7064, 11.1356) construction
  line L382 (35.7064, 11.1356) -> (35.2719, 11.5701) construction
  line L383 (35.2719, 11.5701) -> (34.7358, 11.5701) construction
  spline S125 degree 3 poles (34.7358, 11.5701) (34.1999, 11.5701) (33.7653, 11.1356) (33.7653, 10.5996) knots 0 0 0 0 1 1 1 1
  line L384 (34.7358, 11.5701) -> (34.1999, 11.5701) construction
  line L385 (34.1999, 11.5701) -> (33.7653, 11.1356) construction
  line L386 (33.7653, 11.1356) -> (33.7653, 10.5996) construction
  spline S126 degree 3 poles (33.7653, 10.5996) (33.7653, 10.0636) (34.1999, 9.629) (34.7358, 9.629) knots 0 0 0 0 1 1 1 1
  line L387 (33.7653, 10.5996) -> (33.7653, 10.0636) construction
  line L388 (33.7653, 10.0636) -> (34.1999, 9.629) construction
  line L389 (34.1999, 9.629) -> (34.7358, 9.629) construction
  spline S127 degree 3 poles (34.7358, 9.629) (35.2719, 9.629) (35.7064, 10.0636) (35.7064, 10.5996) knots 0 0 0 0 1 1 1 1
  line L390 (34.7358, 9.629) -> (35.2719, 9.629) construction
  line L391 (35.2719, 9.629) -> (35.7064, 10.0636) construction
  line L392 (35.7064, 10.0636) -> (35.7064, 10.5996) construction
  spline S128 degree 3 poles (38.2606, 10.5996) (38.2606, 11.1356) (37.826, 11.5701) (37.29, 11.5701) knots 0 0 0 0 1 1 1 1
  line L393 (38.2606, 10.5996) -> (38.2606, 11.1356) construction
  line L394 (38.2606, 11.1356) -> (37.826, 11.5701) construction
  line L395 (37.826, 11.5701) -> (37.29, 11.5701) construction
  spline S129 degree 3 poles (37.29, 11.5701) (36.754, 11.5701) (36.3194, 11.1356) (36.3194, 10.5996) knots 0 0 0 0 1 1 1 1
  line L396 (37.29, 11.5701) -> (36.754, 11.5701) construction
  line L397 (36.754, 11.5701) -> (36.3194, 11.1356) construction
  line L398 (36.3194, 11.1356) -> (36.3194, 10.5996) construction
  spline S130 degree 3 poles (36.3194, 10.5996) (36.3194, 10.0636) (36.754, 9.629) (37.29, 9.629) knots 0 0 0 0 1 1 1 1
  line L399 (36.3194, 10.5996) -> (36.3194, 10.0636) construction
  line L400 (36.3194, 10.0636) -> (36.754, 9.629) construction
  line L401 (36.754, 9.629) -> (37.29, 9.629) construction
  spline S131 degree 3 poles (37.29, 9.629) (37.826, 9.629) (38.2606, 10.0636) (38.2606, 10.5996) knots 0 0 0 0 1 1 1 1
  line L402 (37.29, 9.629) -> (37.826, 9.629) construction
  line L403 (37.826, 9.629) -> (38.2606, 10.0636) construction
  line L404 (38.2606, 10.0636) -> (38.2606, 10.5996) construction
  spline S132 degree 3 poles (35.7064, 13.1537) (35.7064, 13.6897) (35.2719, 14.1242) (34.7358, 14.1242) knots 0 0 0 0 1 1 1 1
  line L405 (35.7064, 13.1537) -> (35.7064, 13.6897) construction
  line L406 (35.7064, 13.6897) -> (35.2719, 14.1242) construction
  line L407 (35.2719, 14.1242) -> (34.7358, 14.1242) construction
  spline S133 degree 3 poles (34.7358, 14.1242) (34.1999, 14.1242) (33.7653, 13.6897) (33.7653, 13.1537) knots 0 0 0 0 1 1 1 1
  line L408 (34.7358, 14.1242) -> (34.1999, 14.1242) construction
  line L409 (34.1999, 14.1242) -> (33.7653, 13.6897) construction
  line L410 (33.7653, 13.6897) -> (33.7653, 13.1537) construction
  spline S134 degree 3 poles (33.7653, 13.1537) (33.7653, 12.6177) (34.1999, 12.1831) (34.7358, 12.1831) knots 0 0 0 0 1 1 1 1
  line L411 (33.7653, 13.1537) -> (33.7653, 12.6177) construction
  line L412 (33.7653, 12.6177) -> (34.1999, 12.1831) construction
  line L413 (34.1999, 12.1831) -> (34.7358, 12.1831) construction
  spline S135 degree 3 poles (34.7358, 12.1831) (35.2719, 12.1831) (35.7064, 12.6177) (35.7064, 13.1537) knots 0 0 0 0 1 1 1 1
  line L414 (34.7358, 12.1831) -> (35.2719, 12.1831) construction
  line L415 (35.2719, 12.1831) -> (35.7064, 12.6177) construction
  line L416 (35.7064, 12.6177) -> (35.7064, 13.1537) construction
  spline S136 degree 3 poles (38.2606, 13.1537) (38.2606, 13.6897) (37.826, 14.1242) (37.29, 14.1242) knots 0 0 0 0 1 1 1 1
  line L417 (38.2606, 13.1537) -> (38.2606, 13.6897) construction
  line L418 (38.2606, 13.6897) -> (37.826, 14.1242) construction
  line L419 (37.826, 14.1242) -> (37.29, 14.1242) construction
  spline S137 degree 3 poles (37.29, 14.1242) (36.754, 14.1242) (36.3194, 13.6897) (36.3194, 13.1537) knots 0 0 0 0 1 1 1 1
  line L420 (37.29, 14.1242) -> (36.754, 14.1242) construction
  line L421 (36.754, 14.1242) -> (36.3194, 13.6897) construction
  line L422 (36.3194, 13.6897) -> (36.3194, 13.1537) construction
  spline S138 degree 3 poles (36.3194, 13.1537) (36.3194, 12.6177) (36.754, 12.1831) (37.29, 12.1831) knots 0 0 0 0 1 1 1 1
  line L423 (36.3194, 13.1537) -> (36.3194, 12.6177) construction
  line L424 (36.3194, 12.6177) -> (36.754, 12.1831) construction
  line L425 (36.754, 12.1831) -> (37.29, 12.1831) construction
  spline S139 degree 3 poles (37.29, 12.1831) (37.826, 12.1831) (38.2606, 12.6177) (38.2606, 13.1537) knots 0 0 0 0 1 1 1 1
  line L426 (37.29, 12.1831) -> (37.826, 12.1831) construction
  line L427 (37.826, 12.1831) -> (38.2606, 12.6177) construction
  line L428 (38.2606, 12.6177) -> (38.2606, 13.1537) construction
  spline S140 degree 3 poles (35.7064, 15.7078) (35.7064, 16.2438) (35.2719, 16.6783) (34.7358, 16.6783) knots 0 0 0 0 1 1 1 1
  line L429 (35.7064, 15.7078) -> (35.7064, 16.2438) construction
  line L430 (35.7064, 16.2438) -> (35.2719, 16.6783) construction
  line L431 (35.2719, 16.6783) -> (34.7358, 16.6783) construction
  spline S141 degree 3 poles (34.7358, 16.6783) (34.1999, 16.6783) (33.7653, 16.2438) (33.7653, 15.7078) knots 0 0 0 0 1 1 1 1
  line L432 (34.7358, 16.6783) -> (34.1999, 16.6783) construction
  line L433 (34.1999, 16.6783) -> (33.7653, 16.2438) construction
  line L434 (33.7653, 16.2438) -> (33.7653, 15.7078) construction
  spline S142 degree 3 poles (33.7653, 15.7078) (33.7653, 15.1718) (34.1999, 14.7372) (34.7358, 14.7372) knots 0 0 0 0 1 1 1 1
  line L435 (33.7653, 15.7078) -> (33.7653, 15.1718) construction
  line L436 (33.7653, 15.1718) -> (34.1999, 14.7372) construction
  line L437 (34.1999, 14.7372) -> (34.7358, 14.7372) construction
  spline S143 degree 3 poles (34.7358, 14.7372) (35.2719, 14.7372) (35.7064, 15.1718) (35.7064, 15.7078) knots 0 0 0 0 1 1 1 1
  line L438 (34.7358, 14.7372) -> (35.2719, 14.7372) construction
  line L439 (35.2719, 14.7372) -> (35.7064, 15.1718) construction
  line L440 (35.7064, 15.1718) -> (35.7064, 15.7078) construction
  spline S144 degree 3 poles (38.2606, 15.7078) (38.2606, 16.2438) (37.826, 16.6783) (37.29, 16.6783) knots 0 0 0 0 1 1 1 1
  line L441 (38.2606, 15.7078) -> (38.2606, 16.2438) construction
  line L442 (38.2606, 16.2438) -> (37.826, 16.6783) construction
  line L443 (37.826, 16.6783) -> (37.29, 16.6783) construction
  spline S145 degree 3 poles (37.29, 16.6783) (36.754, 16.6783) (36.3194, 16.2438) (36.3194, 15.7078) knots 0 0 0 0 1 1 1 1
  line L444 (37.29, 16.6783) -> (36.754, 16.6783) construction
  line L445 (36.754, 16.6783) -> (36.3194, 16.2438) construction
  line L446 (36.3194, 16.2438) -> (36.3194, 15.7078) construction
  spline S146 degree 3 poles (36.3194, 15.7078) (36.3194, 15.1718) (36.754, 14.7372) (37.29, 14.7372) knots 0 0 0 0 1 1 1 1
  line L447 (36.3194, 15.7078) -> (36.3194, 15.1718) construction
  line L448 (36.3194, 15.1718) -> (36.754, 14.7372) construction
  line L449 (36.754, 14.7372) -> (37.29, 14.7372) construction
  spline S147 degree 3 poles (37.29, 14.7372) (37.826, 14.7372) (38.2606, 15.1718) (38.2606, 15.7078) knots 0 0 0 0 1 1 1 1
  line L450 (37.29, 14.7372) -> (37.826, 14.7372) construction
  line L451 (37.826, 14.7372) -> (38.2606, 15.1718) construction
  line L452 (38.2606, 15.1718) -> (38.2606, 15.7078) construction
  spline S148 degree 3 poles (35.7064, 18.2619) (35.7064, 18.7979) (35.2719, 19.2324) (34.7358, 19.2324) knots 0 0 0 0 1 1 1 1
  line L453 (35.7064, 18.2619) -> (35.7064, 18.7979) construction
  line L454 (35.7064, 18.7979) -> (35.2719, 19.2324) construction
  line L455 (35.2719, 19.2324) -> (34.7358, 19.2324) construction
  spline S149 degree 3 poles (34.7358, 19.2324) (34.1999, 19.2324) (33.7653, 18.7979) (33.7653, 18.2619) knots 0 0 0 0 1 1 1 1
  line L456 (34.7358, 19.2324) -> (34.1999, 19.2324) construction
  line L457 (34.1999, 19.2324) -> (33.7653, 18.7979) construction
  line L458 (33.7653, 18.7979) -> (33.7653, 18.2619) construction
  spline S150 degree 3 poles (33.7653, 18.2619) (33.7653, 17.7259) (34.1999, 17.2914) (34.7358, 17.2914) knots 0 0 0 0 1 1 1 1
  line L459 (33.7653, 18.2619) -> (33.7653, 17.7259) construction
  line L460 (33.7653, 17.7259) -> (34.1999, 17.2914) construction
  line L461 (34.1999, 17.2914) -> (34.7358, 17.2914) construction
  spline S151 degree 3 poles (34.7358, 17.2914) (35.2719, 17.2914) (35.7064, 17.7259) (35.7064, 18.2619) knots 0 0 0 0 1 1 1 1
  line L462 (34.7358, 17.2914) -> (35.2719, 17.2914) construction
  line L463 (35.2719, 17.2914) -> (35.7064, 17.7259) construction
  line L464 (35.7064, 17.7259) -> (35.7064, 18.2619) construction
  spline S152 degree 3 poles (38.2606, 18.2619) (38.2606, 18.7979) (37.826, 19.2324) (37.29, 19.2324) knots 0 0 0 0 1 1 1 1
  line L465 (38.2606, 18.2619) -> (38.2606, 18.7979) construction
  line L466 (38.2606, 18.7979) -> (37.826, 19.2324) construction
  line L467 (37.826, 19.2324) -> (37.29, 19.2324) construction
  spline S153 degree 3 poles (37.29, 19.2324) (36.754, 19.2324) (36.3194, 18.7979) (36.3194, 18.2619) knots 0 0 0 0 1 1 1 1
  line L468 (37.29, 19.2324) -> (36.754, 19.2324) construction